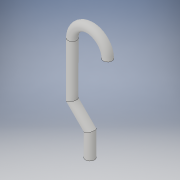
# Autodesk Inventor part: Part9
Saved by Autodesk Inventor 2019.1 (Build 231200000, 200)
## iProperties
Created: 2018-09-18
Part Number: Part9
Material: Generic
Document SubType Name: Modeling
Designer: drawing
Density: 1 g/cm^3
Appearance: Default
Author: drawing
Autodesk Inventor part; units mm, degrees
ref_plane "YZ Plane" through (0, 0, 0) normal (1, 0, 0) x (0, 1, 0)
ref_plane "XZ Plane" through (0, 0, 0) normal (0, 1, 0) x (-1, 0, 0)
ref_plane "XY Plane" through (0, 0, 0) normal (0, 0, 1) x (1, 0, 0)
sketch "Sketch1" plane through (0, 0, 0) normal (0, 0, 1) x (1, 0, 0)
  arc A0 (19.05, 101.6) -> (-19.05, 101.6) centre (0, 101.6) ccw
  line L0 (-19.05, 101.6) -> (-19.05, 44.45)
  line L1 (-19.05, 44.45) -> (0, 25.4)
  line L2 (0, 25.4) -> (0, 0)
  dimension "d1" = 19.05
  dimension "d2" = 45
  dimension "d5" = 25.4
  dimension "d6" = 101.6
  constraints: 7 end point, 2 horizontal alignment, 2 point on circle, 1 centre point, 1 parallel, 1 vertical, 1 vertical alignment
  measures "d1" radius of A0
  measures "d2" angle of L1 L2
  measures "d5" distance of L1.end L2.end
  measures "d6" distance of L2.end A0.centre
sketch "Sketch2" plane through (0, 0, 0) normal (0, 1, 0) x (-1, 0, 0)
  circle A0 centre (0, 0) radius 4.7625
  dimension "d7" = 9.525
  constraints: 1 centre point, 1 coincident
  measures "d7" diameter of A0
sweep "Sweep1" add profiles "Sketch2" path "Sketch1"
sketch "Sketch3" plane through (0, 0, 0) normal (0, -1, 0) x (1, 0, 0)
  point P0 (0, 0)
  point P1 (0, 0)
  constraints: 1 coincident
hole "Hole1" at (0, 0, 0) direction (0, 1, 0) diameter 4.9784 depth 19.05 tip angle 118
body "Solid1"
